Autodesk Fusion 360 part; units mm, degrees
(part 2 of 2)
  ellipse E90 centre (-2.2927, -1.0013) end of major axis (-2.3117, -0.984) minor radius 0.0239 (-2.2684, -0.9976) -> (-2.2679, -1.0045) cw
  line L29 (-2.2679, -1.0045) -> (-2.2733, -1.15)
  ellipse E91 centre (-2.4374, -1.1585) end of major axis (-2.5308, -1.3078) minor radius 0.1594 (-2.2733, -1.15) -> (-2.2759, -1.1743) cw
  spline S246 degree 3 poles (-2.2759, -1.1743) (-2.2803, -1.1894) (-2.2833, -1.226) (-2.2807, -1.2459) knots 0 0 0 0 1 1 1 1
  spline S247 degree 2 poles (-2.2807, -1.2459) (-2.272, -1.3146) (-2.2809, -1.3714) knots 0 0 0 1 1 1
  ellipse E92 centre (-2.1615, -1.3938) end of major axis (-2.2454, -1.3037) minor radius 0.1188 (-2.2815, -1.4035) -> (-2.2809, -1.3714) cw
  spline S248 degree 2 poles (-2.2815, -1.4035) (-2.2772, -1.4387) (-2.2689, -1.4997) knots 0 0 0 1 1 1
  spline S249 degree 3 poles (-2.2689, -1.4997) (-2.2639, -1.5356) (-2.2685, -1.5529) (-2.2732, -1.5955) knots 0 0 0 0 1 1 1 1
  ellipse E93 centre (-2.1916, -1.6067) end of major axis (-2.2507, -1.548) minor radius 0.0809 (-2.2728, -1.6161) -> (-2.2732, -1.5955) cw
  spline S250 degree 2 poles (-2.2728, -1.6161) (-2.2595, -1.711) (-2.2374, -1.8371) knots 0 0 0 1 1 1
  spline S251 degree 2 poles (-2.2374, -1.8371) (-2.2305, -1.8774) (-2.204, -1.9508) knots 0 0 0 1 1 1
  spline S252 degree 2 poles (-2.204, -1.9508) (-2.1785, -2.0218) (-2.1763, -2.0986) knots 0 0 0 1 1 1
  spline S253 degree 3 poles (-2.1763, -2.0986) (-2.1752, -2.1439) (-2.1755, -2.1826) (-2.1677, -2.2277) knots 0 0 0 0 1 1 1 1
  spline S254 degree 2 poles (-2.1677, -2.2277) (-2.1513, -2.3239) (-2.0571, -2.8599) knots 0 0 0 1 1 1
  spline S255 degree 2 poles (-2.0571, -2.8599) (-2.037, -2.9749) (-2.0468, -3.0478) knots 0 0 0 1 1 1
  ellipse E94 centre (-1.9953, -3.0578) end of major axis (-2.0317, -3.0191) minor radius 0.051 (-2.0469, -3.0627) -> (-2.0468, -3.0478) cw
  spline S256 degree 2 poles (-2.0469, -3.0627) (-2.0291, -3.1968) (-2.0135, -3.2586) knots 0 0 0 1 1 1
  spline S257 degree 2 poles (-2.0135, -3.2586) (-1.9918, -3.345) (-1.9145, -3.3679) knots 0 0 0 1 1 1
  spline S258 degree 3 poles (-1.9145, -3.3679) (-1.8879, -3.3758) (-1.8266, -3.3627) (-1.8022, -3.3579) knots 0 0 0 0 1 1 1 1
  spline S259 degree 3 poles (-1.8022, -3.3579) (-1.734, -3.3446) (-1.6593, -3.3588) (-1.5907, -3.3465) knots 0 0 0 0 1 1 1 1
  spline S260 degree 2 poles (-1.5907, -3.3465) (-1.4494, -3.3214) (-1.4474, -3.3211) knots 0 0 0 1 1 1
  spline S261 degree 3 poles (-1.4474, -3.3211) (-1.3177, -3.2964) (-1.2074, -3.3361) (-1.0877, -3.3827) knots 0 0 0 0 1 1 1 1
  spline S262 degree 3 poles (-1.0877, -3.3827) (-1.0295, -3.4053) (-0.9629, -3.4019) (-0.9034, -3.4048) knots 0 0 0 0 1 1 1 1
  ellipse E95 centre (-0.8799, -2.9878) end of major axis (-1.1607, -3.2996) minor radius 0.4148 (-0.8184, -3.3999) -> (-0.9034, -3.4048) cw
  line L30 (-0.8184, -3.3999) -> (-0.5402, -3.3552)
  ellipse E96 centre (-0.5441, -3.3014) end of major axis (-0.5742, -3.348) minor radius 0.0515 (-0.5296, -3.3526) -> (-0.5402, -3.3552) cw
extrude "Extrude3" add sketch "Sketch5" along normal blind 0.8 contours S0 S1 S2 S3 E0 S4 S5 E1 L4 E2 S6 S7 S8 E3 S9 S10 S11 E4 L5 E5 S12 S13 S14 S15 S16 E6 S17 S18 S19 E7 L6 E8 L7 E9 S20 S21 S22 S23 E10 S24 S25 S26 S27 S28 E11 L8 E12 L9 E13 S29 S30 S31 S32 S33 S34 E14 S35 S36 E15 S37 S38 E16 S39 S40 E17 S41 S42 E18 S43 S44 S45 E19 S46 S47 S48 S49 E20 S50 E21 S51 S52 E22 S53 S54 S55 S56 S57 S58 S59 S60 S61 E23 S62 S63 S64 E24 S65 S66 S67 E25 S68 S69 S70 S71 S72 S73 S74 S75 E26 L10 E27 S76 S77 S78 E28 S79 S80 E29 S81 E30 L11 E31 S82 S83 S84 E32 S85 S86 S87 S88 E33 S89 S90 E34 S91 S92 S93 S94 E35 L12 E36 S95 S96 S97 S98 E37 S99 S100 E38 S101 S102 S103 S104 E39 S105 S106 S107 S108 E40 L13 E41 S109 S110 E42 S111 S112 S113 S114 S115 S116 S117 S118 E43 S119 S120 E44 L14 E45 S121 S122 S123 S124 S125 E46 S126 S127 E47 S128 S129 E48 L15 E49 S130 S131 S132 S133 S134 E50 | L16 E51 L17 E52 L18 E53 S135 S136 S137 S138 S139 S140 E54 L19 E55 S141 S142 S143 S144 E56 L20 E57 S145 S146 E58 S147 S148 E59 S149 S150 E60 S151 S152 S153 S154 S155 S156 S157 E61 S158 S159 E62 S160 E63 S161 S162 E64 S163 S164 S165 S166 S167 S168 S169 S170 S171 S172 E65 S173 E66 S174 S175 E67 L21 E68 S176 S177 S178 S179 S180 S181 S182 S183 S184 E69 S185 S186 E70 S187 E71 S188 S189 S190 S191 S192 S193 S194 S195 S196 S197 S198 S199 S200 E72 S201 S202 S203 S204 E73 S205 S206 S207 S208 E74 S209 S210 S211 E75 S212 S213 S214 S215 E76 | S216 S217 S218 S219 S220 S221 S222 S223 E77 L22 E78 L23 E79 L24 E80 S224 S225 S226 E81 L25 E82 L26 E83 L27 E84 S227 S228 S229 E85 S230 S231 E86 L28 S232 S233 S234 S235 E88 S236 S237 S238 S239 S240 S241 S242 S243 S244 E89 S245 E90 L29 E91 S246 S247 E92 S248 S249 E93 S250 S251 S252 S253 S254 S255 E94 S256 S257 S258 S259 S260 S261 S262 E95 L30 E96 | E87
sketch "Sketch6" plane through (0, 0, 3) normal (0, 0, 1) x (-1, 0, 0)
  spline S0 degree 2 poles (-1.4157, -4.7014) (-1.2135, -4.666) (-0.8215, -4.5958) knots 0 0 0 1 1 1
  spline S1 degree 3 poles (-0.8215, -4.5958) (-0.7493, -4.5829) (-0.6698, -4.5863) (-0.6101, -4.6097) knots 0 0 0 0 1 1 1 1
  spline S2 degree 2 poles (-0.6101, -4.6097) (-0.4863, -4.6584) (-0.4774, -4.6609) knots 0 0 0 1 1 1
  spline S3 degree 2 poles (-0.4774, -4.6609) (-0.3743, -4.689) (-0.246, -4.6589) knots 0 0 0 1 1 1
  ellipse E0 centre (-0.24, -4.6668) end of major axis (-0.2497, -4.6618) minor radius 0.0074 (-0.2429, -4.6585) -> (-0.246, -4.6589) ccw
  line L0 (-0.2429, -4.6585) -> (-0.1268, -4.6633)
  ellipse E1 centre (-0.1233, -4.6145) end of major axis (-0.1565, -4.6513) minor radius 0.048 (-0.1268, -4.6633) -> (-0.1164, -4.6626) ccw
  line L1 (-0.1164, -4.6626) -> (0.178, -4.6107)
  ellipse E2 centre (0.1745, -4.5712) end of major axis (0.1525, -4.6059) minor radius 0.0376 (0.178, -4.6107) -> (0.1848, -4.6089) ccw
  line L2 (0.1848, -4.6089) -> (0.3598, -4.5446)
  ellipse E3 centre (0.3425, -4.5175) end of major axis (0.3079, -4.5089) minor radius 0.0292 (0.3598, -4.5446) -> (0.3641, -4.5425) ccw
  spline S4 degree 3 poles (0.3641, -4.5425) (0.3995, -4.5216) (0.4254, -4.5083) (0.4522, -4.4867) knots 0 0 0 0 1 1 1 1
  spline S5 degree 2 poles (0.4522, -4.4867) (0.5599, -4.4003) (0.7494, -4.2762) knots 0 0 0 1 1 1
  spline S6 degree 2 poles (0.7494, -4.2762) (0.7796, -4.2564) (0.8197, -4.2074) knots 0 0 0 1 1 1
  spline S7 degree 3 poles (0.8197, -4.2074) (0.9121, -4.0945) (0.9814, -3.977) (1.0208, -3.8413) knots 0 0 0 0 1 1 1 1
  spline S8 degree 2 poles (1.0208, -3.8413) (1.03, -3.8093) (1.0174, -3.7503) knots 0 0 0 1 1 1
  spline S9 degree 2 poles (1.0174, -3.7503) (1.0003, -3.6721) (1.0042, -3.5823) knots 0 0 0 1 1 1
  ellipse E4 centre (0.9262, -3.5797) end of major axis (0.8743, -3.6384) minor radius 0.0778 (1.0042, -3.5823) -> (1.0033, -3.5673) ccw
  line L3 (1.0033, -3.5673) -> (0.8623, -2.6881)
  ellipse E5 centre (0.8919, -2.6805) end of major axis (0.8707, -2.7036) minor radius 0.0289 (0.8623, -2.6778) -> (0.8623, -2.6881) ccw
  spline S10 degree 2 poles (0.8623, -2.6778) (0.874, -2.6089) (0.8651, -2.5605) knots 0 0 0 1 1 1
  spline S11 degree 3 poles (0.8651, -2.5605) (0.8568, -2.5145) (0.874, -2.4657) (0.8691, -2.4243) knots 0 0 0 0 1 1 1 1
  spline S12 degree 2 poles (0.8691, -2.4243) (0.8646, -2.386) (0.8713, -2.3224) knots 0 0 0 1 1 1
  spline S13 degree 2 poles (0.8713, -2.3224) (0.8755, -2.2838) (0.8639, -2.2083) knots 0 0 0 1 1 1
  ellipse E6 centre (0.9233, -2.2) end of major axis (0.8798, -2.158) minor radius 0.0595 (0.8635, -2.193) -> (0.8639, -2.2083) ccw
  line L4 (0.8635, -2.193) -> (0.8716, -2.1105)
  ellipse E7 centre (0.8645, -2.1085) end of major axis (0.859, -2.103) minor radius 0.0067 (0.8716, -2.1105) -> (0.8714, -2.1074) ccw
  spline S14 degree 2 poles (0.8714, -2.1074) (0.8584, -2.0445) (0.8635, -1.9957) knots 0 0 0 1 1 1
  spline S15 degree 3 poles (0.8635, -1.9957) (0.8724, -1.9123) (0.8579, -1.8552) (0.8429, -1.7689) knots 0 0 0 0 1 1 1 1
  ellipse E8 centre (1.0207, -1.7339) end of major axis (0.899, -1.87) minor radius 0.179 (0.8407, -1.7226) -> (0.8429, -1.7689) ccw
  spline S16 degree 2 poles (0.8407, -1.7226) (0.8484, -1.6337) (0.8381, -1.5795) knots 0 0 0 1 1 1
  spline S17 degree 2 poles (0.8381, -1.5795) (0.8276, -1.5233) (0.7594, -1.1282) knots 0 0 0 1 1 1
  ellipse E9 centre (0.9686, -1.0926) end of major axis (0.8105, -0.9498) minor radius 0.2117 (0.7567, -1.0767) -> (0.7594, -1.1282) ccw
  spline S18 degree 2 poles (0.7567, -1.0767) (0.7629, -0.9856) (0.7454, -0.8864) knots 0 0 0 1 1 1
  spline S19 degree 2 poles (0.7454, -0.8864) (0.3063, 1.6024) (0.2939, 1.676) knots 0 0 0 1 1 1
  ellipse E10 centre (0.5232, 1.7345) end of major axis (0.3744, 1.54) minor radius 0.2249 (0.2908, 1.7116) -> (0.2939, 1.676) ccw
  spline S20 degree 2 poles (0.2908, 1.7116) (0.2898, 1.8399) (0.2831, 1.8718) knots 0 0 0 1 1 1
  spline S21 degree 2 poles (0.2831, 1.8718) (0.2389, 2.079) (0.162, 2.4861) knots 0 0 0 1 1 1
  spline S22 degree 2 poles (0.162, 2.4861) (0.1513, 2.5431) (0.142, 2.6151) knots 0 0 0 1 1 1
  spline S23 degree 2 poles (0.142, 2.6151) (0.1364, 2.6583) (0.1246, 2.7444) knots 0 0 0 1 1 1
  spline S24 degree 2 poles (0.1246, 2.7444) (0.0818, 3.0612) (-0.0439, 3.7455) knots 0 0 0 1 1 1
  spline S25 degree 2 poles (-0.0439, 3.7455) (-0.0481, 3.7681) (-0.0742, 3.8277) knots 0 0 0 1 1 1
  spline S26 degree 3 poles (-0.0742, 3.8277) (-0.1065, 3.9016) (-0.1074, 3.9501) (-0.1273, 4.0596) knots 0 0 0 0 1 1 1 1
  ellipse E11 centre (-0.2332, 4.0352) end of major axis (-0.2818, 3.935) minor radius 0.1069 (-0.1273, 4.0596) -> (-0.1359, 4.0861) ccw
  spline S27 degree 3 poles (-0.1359, 4.0861) (-0.18, 4.1782) (-0.2372, 4.2744) (-0.3262, 4.3521) knots 0 0 0 0 1 1 1 1
  spline S28 degree 2 poles (-0.3262, 4.3521) (-0.3611, 4.3824) (-0.4548, 4.4769) knots 0 0 0 1 1 1
  ellipse E12 centre (-0.5415, 4.3921) end of major axis (-0.6621, 4.3773) minor radius 0.1209 (-0.4548, 4.4769) -> (-0.4796, 4.4962) ccw
  spline S29 degree 2 poles (-0.4796, 4.4962) (-0.6213, 4.5807) (-0.7023, 4.6548) knots 0 0 0 1 1 1
  ellipse E13 centre (-0.8094, 4.5359) end of major axis (-0.8431, 4.6931) minor radius 0.1595 (-0.7023, 4.6548) -> (-0.7458, 4.6831) ccw
  spline S30 degree 2 poles (-0.7458, 4.6831) (-0.843, 4.726) (-0.9509, 4.8047) knots 0 0 0 1 1 1
  spline S31 degree 3 poles (-0.9509, 4.8047) (-1.0484, 4.8759) (-1.1751, 4.884) (-1.2879, 4.906) knots 0 0 0 0 1 1 1 1
  ellipse E14 centre (-1.2277, 5.2287) end of major axis (-1.3866, 5.5178) minor radius 0.326 (-1.3455, 4.9231) -> (-1.2879, 4.906) ccw
  spline S32 degree 3 poles (-1.3455, 4.9231) (-1.4546, 4.9671) (-1.6108, 5.0143) (-1.7181, 5.0027) knots 0 0 0 0 1 1 1 1
  spline S33 degree 2 poles (-1.7181, 5.0027) (-1.7706, 4.9971) (-1.8543, 4.9802) knots 0 0 0 1 1 1
  spline S34 degree 2 poles (-1.8543, 4.9802) (-1.8782, 4.9753) (-1.9619, 4.9759) knots 0 0 0 1 1 1
  spline S35 degree 3 poles (-1.9619, 4.9759) (-2.0499, 4.9764) (-2.17, 4.9524) (-2.2256, 4.9415) knots 0 0 0 0 1 1 1 1
  spline S36 degree 3 poles (-2.2256, 4.9415) (-2.3063, 4.9258) (-2.4169, 4.9327) (-2.4735, 4.9589) knots 0 0 0 0 1 1 1 1
  spline S37 degree 3 poles (-2.4735, 4.9589) (-2.598, 5.0164) (-2.7075, 5.025) (-2.843, 4.9972) knots 0 0 0 0 1 1 1 1
  spline S38 degree 2 poles (-2.843, 4.9972) (-2.8781, 4.99) (-2.987, 4.9902) knots 0 0 0 1 1 1
  spline S39 degree 2 poles (-2.987, 4.9902) (-3.0182, 4.9903) (-3.0474, 4.9859) knots 0 0 0 1 1 1
  spline S40 degree 2 poles (-3.0474, 4.9859) (-3.1024, 4.9779) (-3.7272, 4.8664) knots 0 0 0 1 1 1
  spline S41 degree 2 poles (-3.7272, 4.8664) (-3.758, 4.861) (-3.8436, 4.826) knots 0 0 0 1 1 1
  ellipse E15 centre (-3.9074, 4.9646) end of major axis (-4.0453, 5.0348) minor radius 0.1493 (-3.8728, 4.8171) -> (-3.8436, 4.826) ccw
  spline S42 degree 3 poles (-3.8728, 4.8171) (-3.9744, 4.7964) (-4.0535, 4.7929) (-4.1401, 4.7137) knots 0 0 0 0 1 1 1 1
  ellipse E16 centre (-4.0936, 4.6607) end of major axis (-4.1066, 4.7305) minor radius 0.0695 (-4.1401, 4.7137) -> (-4.1587, 4.686) ccw
  spline S43 degree 3 poles (-4.1587, 4.686) (-4.1691, 4.6578) (-4.1835, 4.6249) (-4.2053, 4.5961) knots 0 0 0 0 1 1 1 1
  spline S44 degree 2 poles (-4.2053, 4.5961) (-4.248, 4.54) (-4.2995, 4.4723) knots 0 0 0 1 1 1
  ellipse E17 centre (-4.1555, 4.3628) end of major axis (-4.329, 4.311) minor radius 0.1809 (-4.2995, 4.4723) -> (-4.3262, 4.4229) ccw
  line L5 (-4.3262, 4.4229) -> (-4.373, 4.29)
  ellipse E18 centre (-4.4432, 4.3186) end of major axis (-4.4661, 4.3932) minor radius 0.0745 (-4.3813, 4.2734) -> (-4.373, 4.29) ccw
  spline S45 degree 3 poles (-4.3813, 4.2734) (-4.4268, 4.2036) (-4.4664, 4.1237) (-4.465, 4.0417) knots 0 0 0 0 1 1 1 1
  spline S46 degree 3 poles (-4.465, 4.0417) (-4.4634, 3.9479) (-4.4738, 3.9099) (-4.4575, 3.8189) knots 0 0 0 0 1 1 1 1
  spline S47 degree 3 poles (-4.4575, 3.8189) (-4.4391, 3.7167) (-4.3939, 3.5036) (-4.3876, 3.3414) knots 0 0 0 0 1 1 1 1
  spline S48 degree 2 poles (-4.3876, 3.3414) (-4.3814, 3.1835) (-4.3338, 3.036) knots 0 0 0 1 1 1
  spline S49 degree 2 poles (-4.3338, 3.036) (-4.2999, 2.9317) (-4.2892, 2.8676) knots 0 0 0 1 1 1
  spline S50 degree 2 poles (-4.2892, 2.8676) (-4.263, 2.7098) (-4.2343, 2.5544) knots 0 0 0 1 1 1
  spline S51 degree 2 poles (-4.2343, 2.5544) (-4.2213, 2.484) (-4.214, 2.3485) knots 0 0 0 1 1 1
  spline S52 degree 2 poles (-4.214, 2.3485) (-4.2073, 2.2219) (-4.1791, 2.0833) knots 0 0 0 1 1 1
  spline S53 degree 2 poles (-4.1791, 2.0833) (-4.166, 2.0193) (-4.0672, 1.4411) knots 0 0 0 1 1 1
  ellipse E19 centre (-4.2448, 1.4073) end of major axis (-4.3682, 1.274) minor radius 0.1791 (-4.0656, 1.3896) -> (-4.0672, 1.4411) ccw
  spline S54 degree 2 poles (-4.0656, 1.3896) (-4.0768, 1.2887) (-4.0895, 1.113) knots 0 0 0 1 1 1
  spline S55 degree 3 poles (-4.0895, 1.113) (-4.0916, 1.0841) (-4.0882, 1.0686) (-4.0838, 1.0306) knots 0 0 0 0 1 1 1 1
  ellipse E20 centre (-4.2689, 1.008) end of major axis (-4.4025, 0.8772) minor radius 0.1857 (-4.0845, 0.9827) -> (-4.0838, 1.0306) ccw
  spline S56 degree 3 poles (-4.0845, 0.9827) (-4.0943, 0.9125) (-4.0835, 0.868) (-4.069, 0.7768) knots 0 0 0 0 1 1 1 1
  ellipse E21 centre (-4.14, 0.7649) end of major axis (-4.1915, 0.7145) minor radius 0.0717 (-4.0694, 0.7518) -> (-4.069, 0.7768) ccw
  spline S57 degree 2 poles (-4.0694, 0.7518) (-4.0811, 0.6881) (-4.0608, 0.5783) knots 0 0 0 1 1 1
  spline S58 degree 2 poles (-4.0608, 0.5783) (-4.0582, 0.5644) (-4.0162, 0.3192) knots 0 0 0 1 1 1
  spline S59 degree 2 poles (-4.0162, 0.3192) (-4.0119, 0.2939) (-4.0146, 0.2342) knots 0 0 0 1 1 1
  spline S60 degree 3 poles (-4.0146, 0.2342) (-4.0169, 0.1862) (-4.0108, 0.1386) (-4.0047, 0.1012) knots 0 0 0 0 1 1 1 1
  spline S61 degree 2 poles (-4.0047, 0.1012) (-3.9862, -0.0128) (-3.9186, -0.3923) knots 0 0 0 1 1 1
  spline S62 degree 2 poles (-3.9186, -0.3923) (-3.905, -0.4688) (-3.9048, -0.553) knots 0 0 0 1 1 1
  spline S63 degree 2 poles (-3.9048, -0.553) (-3.9044, -0.6385) (-3.8784, -0.7852) knots 0 0 0 1 1 1
  spline S64 degree 2 poles (-3.8784, -0.7852) (-3.8704, -0.8294) (-3.8189, -1.1194) knots 0 0 0 1 1 1
  spline S65 degree 2 poles (-3.8189, -1.1194) (-3.7984, -1.2348) (-3.7802, -1.4169) knots 0 0 0 1 1 1
  spline S66 degree 2 poles (-3.7802, -1.4169) (-3.7643, -1.5766) (-3.7414, -1.7147) knots 0 0 0 1 1 1
  spline S67 degree 2 poles (-3.7414, -1.7147) (-3.6783, -2.0981) (-3.4693, -3.2411) knots 0 0 0 1 1 1
  spline S68 degree 3 poles (-3.4693, -3.2411) (-3.456, -3.3139) (-3.4163, -3.4049) (-3.4027, -3.4828) knots 0 0 0 0 1 1 1 1
  spline S69 degree 2 poles (-3.4027, -3.4828) (-3.3844, -3.5875) (-3.3465, -3.8069) knots 0 0 0 1 1 1
  ellipse E22 centre (-3.249, -3.7891) end of major axis (-3.2942, -3.8786) minor radius 0.0986 (-3.3465, -3.8069) -> (-3.3378, -3.8343) ccw
  spline S70 degree 2 poles (-3.3378, -3.8343) (-3.2562, -4.003) (-3.1644, -4.0883) knots 0 0 0 1 1 1
  spline S71 degree 2 poles (-3.1644, -4.0883) (-3.097, -4.1509) (-3.0128, -4.2269) knots 0 0 0 1 1 1
  spline S72 degree 2 poles (-3.0128, -4.2269) (-2.9673, -4.2679) (-2.9153, -4.2969) knots 0 0 0 1 1 1
  spline S73 degree 2 poles (-2.9153, -4.2969) (-2.8253, -4.347) (-2.7552, -4.4201) knots 0 0 0 1 1 1
  ellipse E23 centre (-2.6593, -4.329) end of major axis (-2.7893, -4.355) minor radius 0.1313 (-2.7552, -4.4201) -> (-2.7074, -4.4516) ccw
  spline S74 degree 2 poles (-2.7074, -4.4516) (-2.638, -4.478) (-2.5579, -4.5341) knots 0 0 0 1 1 1
  spline S75 degree 3 poles (-2.5579, -4.5341) (-2.5012, -4.5736) (-2.4501, -4.5935) (-2.3918, -4.6055) knots 0 0 0 0 1 1 1 1
  spline S76 degree 2 poles (-2.3918, -4.6055) (-2.2724, -4.6301) (-2.1771, -4.6185) knots 0 0 0 1 1 1
  spline S77 degree 3 poles (-2.1771, -4.6185) (-2.1067, -4.61) (-2.0542, -4.6242) (-1.983, -4.6131) knots 0 0 0 0 1 1 1 1
  ellipse E24 centre (-1.9617, -4.7283) end of major axis (-2.0428, -4.6426) minor radius 0.1152 (-1.9368, -4.6149) -> (-1.983, -4.6131) ccw
  spline S78 degree 2 poles (-1.9368, -4.6149) (-1.8356, -4.6393) (-1.7527, -4.6682) knots 0 0 0 1 1 1
  spline S79 degree 2 poles (-1.7527, -4.6682) (-1.6664, -4.6985) (-1.6077, -4.6995) knots 0 0 0 1 1 1
  spline S80 degree 2 poles (-1.6077, -4.6995) (-1.5089, -4.7013) (-1.457, -4.7039) knots 0 0 0 1 1 1
  ellipse E25 centre (-1.4417, -4.5075) end of major axis (-1.5763, -4.6549) minor radius 0.1929 (-1.457, -4.7039) -> (-1.4157, -4.7014) ccw
  line L6 (-0.3524, -3.26) -> (-1.2616, 3.6153)
  line L7 (-1.2616, 3.6153) -> (-3.1486, 3.6153)
  line L8 (-3.1486, 3.6153) -> (-2.1853, -3.6684)
  line L9 (-0.3524, -3.26) -> (-2.2393, -3.26)
  constraint horizontal L7
  constraint parallel L6 L8
  constraint coincident L8 L9.end
  constraint horizontal L9
extrude "Extrude4" cut sketch "Sketch6" against normal blind 0.8 contours L6 L7 L8 L9
fillet "Fillet2" radius 0.25 4 edges at (0.3524, 3.26, 2.6) (2.2393, 3.26, 2.6) (3.1486, -3.6153, 2.6) (1.2616, -3.6153, 2.6)
